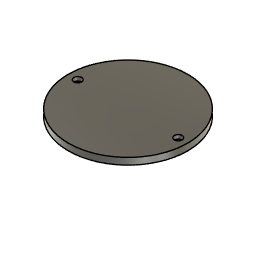
teline rungon pohjaan v1 (Autodesk Fusion 360 design; units mm, degrees)
Autodesk Fusion 360 part; units mm, degrees
sketch "Sketch1" plane through (0, 0, 0) normal (0, 0, 1) x (1, 0, 0)
  circle A0 centre (0, 0) radius 26.7785
  line L0 (0, 0) -> (-26.7785, 0) construction
  line L1 (0, 0) -> (26.7785, 0) construction
  circle A1 centre (-22.5285, 0) radius 3
  circle A2 centre (-22.5285, 0) radius 1.75
  circle A3 centre (22.5285, 0) radius 3
  circle A4 centre (22.5285, 0) radius 1.75
  circle A5 centre (0, 0) radius 4
  dimension "d1" = 53.557
  dimension "d2" = 6
  dimension "d3" = 3.5
  dimension "d4" = 4.25
  dimension "d5" = 6
  dimension "d6" = 3.5
  dimension "d8" = 4.25
  dimension "d12" = 8
  constraint coincident A0.centre L0.start
  constraint coincident A0 L0.end
  constraint horizontal L0
  constraint coincident A0 L1.end
  constraint parallel L0 L1
  constraint coincident L0 A1.centre
  constraint concentric A1 A2
  constraint concentric A3 A4
  constraint coincident L1 A3.centre
  measures "d1" diameter of A0
  measures "d2" diameter of A1
  measures "d3" diameter of A2
  measures "d4" distance of L0.end A1.centre
  measures "d5" diameter of A3
  measures "d6" diameter of A4
  measures "d8" distance of L1.end A3.centre
  measures "d12" diameter of A5
extrude "Extrude1" add sketch "Sketch1" along normal blind 3 contours A0 | A1 | A3 | A5
chamfer "Chamfer1" distance 1.25 angle 45 2 edges at (20.8969, 0.6328, 0) (-24.1601, 0.6328, 0)
extrude "Extrude2" add sketch "Sketch1" against normal blind 12 contours A5
fillet "Fillet1" radius 3 1 edges at (-3.7293, -1.4465, 0)
